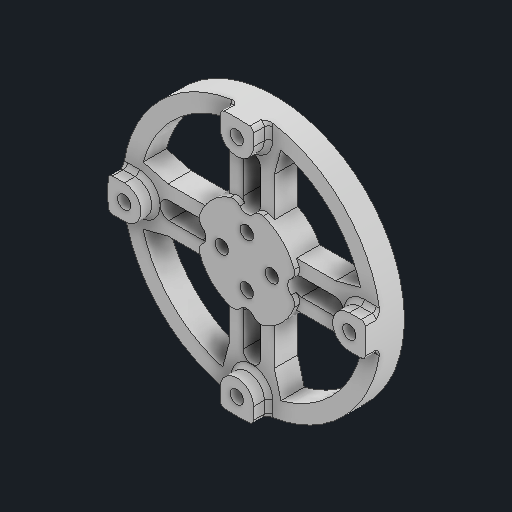
# Autodesk Inventor part: Rotator_B
Saved by Autodesk Inventor 2025.1 (Build 291241020, 241B)
## iProperties
Created: 2025-07-24
Part Number: Rotator_B
Material: 일반
Document SubType Name: Modeling
Designer: acalo
Density: 1 g/cm^3
Appearance: 기본값
Author: acalo
Autodesk Inventor part; units mm, degrees
ref_plane "YZ Plane" through (0, 0, 0) normal (1, 0, 0) x (0, 1, 0)
ref_plane "XZ Plane" through (0, 0, 0) normal (0, 1, 0) x (-1, 0, 0)
ref_plane "XY Plane" through (0, 0, 0) normal (0, 0, 1) x (1, 0, 0)
sketch "스케치1" plane through (0, 0, 0) normal (0, 0, 1) x (1, 0, 0)
  circle A0 centre (27, 0) radius 1.65
  circle A1 centre (0, 0) radius 31
  line L0 (5.4, 20.1531) -> (6.9881, 26.08)
  line L1 (20.1531, 5.4) -> (26.08, 6.9881)
  arc A2 (26.08, 6.9881) -> (6.9881, 26.08) centre (0, 0) ccw
  circle A3 centre (-4.8, 0) radius 1.65
  circle A4 centre (4.8, 0) radius 1.65
  line L2 (-5.4, 20.1531) -> (-6.9881, 26.08)
  line L3 (-20.1531, 5.4) -> (-26.08, 6.9881)
  arc A5 (-6.9881, 26.08) -> (-26.08, 6.9881) centre (0, 0) ccw
  line L4 (5.4, -20.1531) -> (6.9881, -26.08)
  line L5 (20.1531, -5.4) -> (26.08, -6.9881)
  arc A6 (6.9881, -26.08) -> (26.08, -6.9881) centre (0, 0) ccw
  line L6 (-20.1531, -5.4) -> (-26.08, -6.9881)
  arc A7 (-26.08, -6.9881) -> (-6.9881, -26.08) centre (0, 0) ccw
  line L7 (-5.4, -20.1531) -> (-6.9881, -26.08)
  line L8 (20.1531, -5.4) -> (8.4167, -5.4)
  line L9 (5.4, -8.4167) -> (5.4, -20.1531)
  line L10 (-5.4, -8.4167) -> (-5.4, -20.1531)
  line L11 (-8.4167, -5.4) -> (-20.1531, -5.4)
  line L12 (-5.4, 20.1531) -> (-5.4, 8.4167)
  line L13 (-8.4167, 5.4) -> (-20.1531, 5.4)
  line L14 (20.1531, 5.4) -> (8.4167, 5.4)
  line L15 (5.4, 20.1531) -> (5.4, 8.4167)
  arc A8 (-5.4, 8.4167) -> (-8.4167, 5.4) centre (0, 0) ccw
  arc A9 (8.4167, 5.4) -> (5.4, 8.4167) centre (0, 0) ccw
  arc A10 (-8.4167, -5.4) -> (-5.4, -8.4167) centre (0, 0) ccw
  arc A11 (5.4, -8.4167) -> (8.4167, -5.4) centre (0, 0) ccw
  circle A12 centre (0, 27) radius 1.65
  circle A13 centre (-27, 0) radius 1.65
  circle A14 centre (0, -27) radius 1.65
  line L16 (-27, 0) -> (-4.8, 0)
  line L17 (-19.9, 0) -> (-11.9, 0) construction
  line L18 (-19.9, -2.1) -> (-11.9, -2.1)
  line L19 (-11.9, 2.1) -> (-19.9, 2.1)
  arc A15 (-19.9, 2.1) -> (-19.9, -2.1) centre (-19.9, 0) ccw
  arc A16 (-11.9, -2.1) -> (-11.9, 2.1) centre (-11.9, 0) ccw
  arc A17 (2.1, -11.9) -> (-2.1, -11.9) centre (0, -11.9) ccw
  line L20 (2.1, -19.9) -> (2.1, -11.9)
  line L21 (0, -19.9) -> (0, -11.9) construction
  line L22 (-2.1, -11.9) -> (-2.1, -19.9)
  line L23 (0, -27) -> (0, -4.8)
  arc A18 (-2.1, -19.9) -> (2.1, -19.9) centre (0, -19.9) ccw
  arc A19 (11.9, 2.1) -> (11.9, -2.1) centre (11.9, 0) ccw
  line L24 (19.9, 2.1) -> (11.9, 2.1)
  line L25 (19.9, 0) -> (11.9, 0) construction
  line L26 (11.9, -2.1) -> (19.9, -2.1)
  line L27 (27, 0) -> (4.8, 0)
  arc A20 (19.9, -2.1) -> (19.9, 2.1) centre (19.9, 0) ccw
  arc A21 (-2.1, 11.9) -> (2.1, 11.9) centre (0, 11.9) ccw
  line L28 (-2.1, 19.9) -> (-2.1, 11.9)
  line L29 (0, 19.9) -> (0, 11.9) construction
  line L30 (2.1, 11.9) -> (2.1, 19.9)
  line L31 (0, 27) -> (0, 4.8)
  arc A22 (2.1, 19.9) -> (-2.1, 19.9) centre (0, 19.9) ccw
  circle A23 centre (0, 0) radius 12
  point P0 (5.9528, 22.2163)
  point P1 (22.2163, 5.9528)
  point P2 (-5.9528, 22.2163)
  point P3 (-22.2163, 5.9528)
  point P4 (5.9528, -22.2163)
  point P5 (22.2163, -5.9528)
  point P6 (-22.2163, -5.9528)
  point P7 (-5.9528, -22.2163)
  point P8 (-15.9, 0)
  point P9 (0, -15.9)
  point P10 (15.9, 0)
  point P11 (0, 15.9)
  point P12 (11.8151, 2.0983)
  point P13 (2.0983, 11.8151)
  point P14 (-2.0983, 11.8151)
  point P15 (-11.8151, 2.0983)
  point P16 (-11.8151, -2.0983)
  point P17 (-2.0983, -11.8151)
  point P18 (2.0983, -11.8151)
  point P19 (11.8151, -2.0983)
  point P20 (5.4, 10.7163)
  point P21 (10.7163, 5.4)
  point P22 (10.7163, -5.4)
  point P23 (5.4, -10.7163)
  point P24 (-5.4, -10.7163)
  point P25 (-10.7163, -5.4)
  point P26 (-10.7163, 5.4)
  point P27 (-5.4, 10.7163)
  dimension "d19" = 3.3
  dimension "d24" = 360
  dimension "d26" = 4
  dimension "d27" = 4.2
  dimension "d30" = 360
  dimension "d32" = 24
  constraints: 72 end point, 32 point on circle, 24 centre point, 12 point on line, 4 tangent, 3 horizontal, 2 coincident, 2 midpoint, 1 parallel, 70 other
  measures "d19" diameter of A4
  measures "d26" distance of point (-15.9, 0) L17.end
  measures "d27" diameter of A16
  measures "d32" diameter of A23
extrude "돌출1" add sketch "스케치1" along normal blind 4.8 contours A23 L14 A9 L15 | L15 A9 L14 A23 A19 L8 A11 L9 A17 L10 A10 L11 A16 L13 A8 L12 A21 | L12 A8 L13 A23 | A23 L9 A11 L8 | L11 A10 L10 A23
extrude "돌출2" add sketch "스케치1" along normal blind 3.6 contours A1
fillet "모깎기1" radius 2 8 edges at (2.0983, 11.8151, 4.2) (-2.0983, 11.8151, 4.2) (-11.8151, 2.0983, 4.2) (-11.8151, -2.0983, 4.2) (-2.0983, -11.8151, 4.2) (2.0983, -11.8151, 4.2) (11.8151, -2.0983, 4.2) (11.8151, 2.0983, 4.2)
sketch "스케치2" plane through (0, 0, 0) normal (0, 0, -1) x (-1, 0, 0)
  arc A0 (-2.1, 11.9) -> (2.1, 11.9) centre (0, 11.9) ccw projected
  line L0 (-2.1, 19.9) -> (-2.1, 11.9) projected
  arc A1 (2.1, 19.9) -> (-2.1, 19.9) centre (0, 19.9) ccw projected
  line L1 (2.1, 11.9) -> (2.1, 19.9) projected
  line L2 (5.4, 20.1531) -> (5.4, 10.7163) projected
  line L3 (6.9881, 26.08) -> (5.4, 20.1531) projected
  arc A2 (26.08, 6.9881) -> (6.9881, 26.08) centre (0, 0) ccw projected
  line L4 (20.1531, 5.4) -> (26.08, 6.9881) projected
  line L5 (10.7163, 5.4) -> (20.1531, 5.4) projected
  arc A3 (10.7163, 5.4) -> (5.4, 10.7163) centre (0, 0) ccw projected
  arc A4 (11.9, 2.1) -> (11.9, -2.1) centre (11.9, 0) ccw projected
  line L6 (19.9, 2.1) -> (11.9, 2.1) projected
  arc A5 (19.9, -2.1) -> (19.9, 2.1) centre (19.9, 0) ccw projected
  line L7 (11.9, -2.1) -> (19.9, -2.1) projected
  line L8 (20.1531, -5.4) -> (10.7163, -5.4) projected
  line L9 (26.08, -6.9881) -> (20.1531, -5.4) projected
  arc A6 (6.9881, -26.08) -> (26.08, -6.9881) centre (0, 0) ccw projected
  line L10 (5.4, -20.1531) -> (6.9881, -26.08) projected
  line L11 (5.4, -10.7163) -> (5.4, -20.1531) projected
  arc A7 (5.4, -10.7163) -> (10.7163, -5.4) centre (0, 0) ccw projected
  arc A8 (2.1, -11.9) -> (-2.1, -11.9) centre (0, -11.9) ccw projected
  line L12 (2.1, -19.9) -> (2.1, -11.9) projected
  arc A9 (-2.1, -19.9) -> (2.1, -19.9) centre (0, -19.9) ccw projected
  line L13 (-2.1, -11.9) -> (-2.1, -19.9) projected
  line L14 (-5.4, -20.1531) -> (-5.4, -10.7163) projected
  line L15 (-6.9881, -26.08) -> (-5.4, -20.1531) projected
  arc A10 (-26.08, -6.9881) -> (-6.9881, -26.08) centre (0, 0) ccw projected
  line L16 (-20.1531, -5.4) -> (-26.08, -6.9881) projected
  line L17 (-10.7163, -5.4) -> (-20.1531, -5.4) projected
  arc A11 (-10.7163, -5.4) -> (-5.4, -10.7163) centre (0, 0) ccw projected
  arc A12 (-11.9, -2.1) -> (-11.9, 2.1) centre (-11.9, 0) ccw projected
  line L18 (-19.9, -2.1) -> (-11.9, -2.1) projected
  arc A13 (-19.9, 2.1) -> (-19.9, -2.1) centre (-19.9, 0) ccw projected
  line L19 (-11.9, 2.1) -> (-19.9, 2.1) projected
  circle A14 centre (-27, 0) radius 1.65 projected
  circle A15 centre (0, -27) radius 1.65 projected
  circle A16 centre (27, 0) radius 1.65 projected
  circle A17 centre (0, 27) radius 1.65 projected
  circle A18 centre (0, 0) radius 31 projected
  line L20 (-20.1531, 5.4) -> (-10.7163, 5.4) projected
  line L21 (-26.08, 6.9881) -> (-20.1531, 5.4) projected
  arc A19 (-6.9881, 26.08) -> (-26.08, 6.9881) centre (0, 0) ccw projected
  line L22 (-5.4, 20.1531) -> (-6.9881, 26.08) projected
  line L23 (-5.4, 10.7163) -> (-5.4, 20.1531) projected
  arc A20 (-5.4, 10.7163) -> (-10.7163, 5.4) centre (0, 0) ccw projected
  circle A21 centre (-4.8, 0) radius 1.65 projected
  circle A22 centre (4.8, 0) radius 1.65 projected
  circle A23 centre (0, -27) radius 2.8
  circle A24 centre (-27, 0) radius 2.8
  circle A25 centre (0, 27) radius 2.8
  circle A26 centre (27, 0) radius 2.8
  dimension "d38" = 5.6
  dimension "d39" = 5.6
  dimension "d40" = 5.6
  dimension "d41" = 5.6
  constraints: 4 centre point, 1 coincident
  measures "d38" diameter of A23
  measures "d39" diameter of A24
  measures "d40" diameter of A25
  measures "d41" diameter of A26
sketch "스케치3" plane through (0, 0, 3.6) normal (0, 0, 1) x (1, 0, 0)
  circle A0 centre (0, -27) radius 1.65 projected
  circle A1 centre (0, 0) radius 31 projected
  arc A2 (4, -27) -> (-4, -27) centre (0, -27) ccw
  line L0 (-4, -27) -> (-4, -30.7409)
  line L1 (0, -27) -> (0, -16.0114)
  line L2 (4, -27) -> (4, -30.7409)
  constraints: 6 end point, 4 point on circle, 3 vertical, 1 centre point, 1 coincident, 1 tangent
extrude "돌출4" add sketch "스케치3" along normal blind 3.6 contours L0 A2 L2 A1 picked at (3.1504, -28.5087)
pattern_circular "원형 패턴1" count 4 over 360 about axis through (0, 0, 0) along (0, 0, 1) of "돌출4"
fillet "모깎기2" radius 1 8 edges at (-4, -30.7409, 5.4) (4, -30.7409, 5.4) (30.7409, -4, 5.4) (30.7409, 4, 5.4) (4, 30.7409, 5.4) (-4, 30.7409, 5.4) (-30.7409, 4, 5.4) (-30.7409, -4, 5.4)
fillet "모깎기3" radius 1 20 edges at (23, 0, 3.6) (28.4248, 4, 3.6) (30.5204, 3.7416, 3.6) (30.5204, -3.7416, 3.6) (28.4248, -4, 3.6) (3.7416, -30.5204, 3.6) (0, -23, 3.6) (-4, -28.4248, 3.6) (-3.7416, -30.5204, 3.6) (4, -28.4248, 3.6) (-4, 28.4248, 3.6) (-3.7416, 30.5204, 3.6) (4, 28.4248, 3.6) (3.7416, 30.5204, 3.6) (0, 23, 3.6) (-28.4248, -4, 3.6) (-30.5204, -3.7416, 3.6) (-28.4248, 4, 3.6) (-30.5204, 3.7416, 3.6) (-23, 0, 3.6)
thicken "두껍게 하기1" operation add thickness 2 both sides no extend neighbours no toward (0, 0, -1) faces at (0.0844, 4.0012, 0)
sketch "스케치4" plane through (0, 0, 4.8) normal (0, 0, 1) x (1, 0, 0)
  circle A0 centre (0, 0) radius 10
  circle A1 centre (4.8, 0) radius 1.65 projected
  circle A2 centre (-4.8, 0) radius 1.65 projected
  line L0 (0, 0) -> (0, 6)
  circle A3 centre (0, 6) radius 1.65
  line L1 (0, 6) -> (0, 8.7)
  line L2 (1.5588, 8.7) -> (3.1177, 6)
  line L3 (3.1177, 6) -> (1.5588, 3.3)
  line L4 (1.5588, 3.3) -> (-1.5588, 3.3)
  line L5 (-1.5588, 3.3) -> (-3.1177, 6)
  line L6 (-3.1177, 6) -> (-1.5588, 8.7)
  line L7 (-1.5588, 8.7) -> (1.5588, 8.7)
  circle A4 centre (-6, 0) radius 1.65
  line L8 (-6, 3.1177) -> (-3.3, 1.5588)
  line L9 (-3.3, 1.5588) -> (-3.3, -1.5588)
  line L10 (-3.3, -1.5588) -> (-6, -3.1177)
  line L11 (-6, -3.1177) -> (-8.7, -1.5588)
  line L12 (-8.7, -1.5588) -> (-8.7, 1.5588)
  line L13 (-8.7, 1.5588) -> (-6, 3.1177)
  circle A5 centre (0, -6) radius 1.65
  line L14 (-3.1177, -6) -> (-1.5588, -3.3)
  line L15 (-1.5588, -3.3) -> (1.5588, -3.3)
  line L16 (1.5588, -3.3) -> (3.1177, -6)
  line L17 (3.1177, -6) -> (1.5588, -8.7)
  line L18 (1.5588, -8.7) -> (-1.5588, -8.7)
  line L19 (-1.5588, -8.7) -> (-3.1177, -6)
  circle A6 centre (6, 0) radius 1.65
  line L20 (6, -3.1177) -> (3.3, -1.5588)
  line L21 (3.3, -1.5588) -> (3.3, 1.5588)
  line L22 (3.3, 1.5588) -> (6, 3.1177)
  line L23 (6, 3.1177) -> (8.7, 1.5588)
  line L24 (8.7, 1.5588) -> (8.7, -1.5588)
  line L25 (8.7, -1.5588) -> (6, -3.1177)
  point P0 (-8.7, 0)
  point P1 (0, -8.7)
  point P2 (8.7, 0)
  point P3 (-3.3, -0.6874)
  point P4 (-3.3, 0.6874)
  dimension "d53" = 20
  dimension "d54" = 6
  dimension "d55" = 3.3
  dimension "d56" = 2.7
  dimension "d59" = 360
  constraints: 52 end point, 5 centre point, 3 coincident, 2 vertical, 1 midpoint, 74 other
  measures "d53" diameter of A0
  measures "d54" distance of L0.start L0.end
  measures "d55" diameter of A3
  measures "d56" distance of L1.start L1.end
extrude "돌출5" add sketch "스케치4" against normal up to surface (6.8 mm away) contours A1 A6 | A6 A1 L21 | L21 A1 | A2 L9 | L9 A2 A4 | A4 A2 picked at (5.0657, -0.1306) picked at (-5.0657, 0.1306)
extrude "돌출6" cut sketch "스케치4" against normal through all contours A1 A6 | A1 A6 | A4 A2 | A2 A4 | A3 L1 L0 | L0 L1 A3 | A5
sketch "스케치5" plane through (0, 0, 4.8) normal (0, 0, 1) x (1, 0, 0)
  circle A0 centre (0, -6) radius 1.65 projected
  circle A1 centre (0, -6) radius 1.6
  point P0 (0, 0)
  dimension "d65" = 3.2
  constraints: 1 centre point, 1 coincident
  measures "d65" diameter of A1
extrude "돌출7" add sketch "스케치5" against normal up to surface (6.8 mm away)
sketch "스케치6" plane through (0, 0, 7.2) normal (0, 0, 1) x (1, 0, 0)
  circle A0 centre (0, -27) radius 1.65 projected
  circle A1 centre (0, -27) radius 1.6
  point P0 (0, 0)
  dimension "d68" = 0.05
  constraints: 1 centre point
  measures "d68" radial gap between concentric circles of A0 A1
extrude "돌출8" add sketch "스케치6" against normal up to surface (9.2 mm away)
pattern_circular "원형 패턴2" count 4 over 360 about axis through (0, 0, 0) along (0, 0, 1) of "돌출7", "돌출8"
sketch "스케치7" plane through (0, 0, -2) normal (0, 0, -1) x (-1, 0, 0)
  circle A0 centre (0, 27) radius 1.6 projected
  circle A1 centre (6, 0) radius 1.6 projected
  circle A2 centre (27, 0) radius 1.6 projected
  circle A3 centre (0, 6) radius 1.6 projected
  circle A4 centre (0, 27) radius 1.6 projected
  circle A5 centre (-6, 0) radius 1.6 projected
  circle A6 centre (-27, 0) radius 1.6 projected
  circle A7 centre (0, -27) radius 1.6 projected
  circle A8 centre (0, -6) radius 1.6 projected
  line L0 (-20.1531, 5.4) -> (-10.7163, 5.4) projected
  line L1 (-26.08, 6.9881) -> (-20.1531, 5.4) projected
  arc A9 (-6.9881, 26.08) -> (-26.08, 6.9881) centre (0, 0) ccw projected
  line L2 (-5.4, 20.1531) -> (-6.9881, 26.08) projected
  line L3 (-5.4, 10.7163) -> (-5.4, 20.1531) projected
  arc A10 (-5.4, 10.7163) -> (-10.7163, 5.4) centre (0, 0) ccw projected
  circle A11 centre (0, 0) radius 31 projected
  arc A12 (-11.9, -2.1) -> (-11.9, 2.1) centre (-11.9, 0) ccw projected
  line L4 (-19.9, -2.1) -> (-11.9, -2.1) projected
  arc A13 (-19.9, 2.1) -> (-19.9, -2.1) centre (-19.9, 0) ccw projected
  line L5 (-11.9, 2.1) -> (-19.9, 2.1) projected
  line L6 (-5.4, -20.1531) -> (-5.4, -10.7163) projected
  line L7 (-6.9881, -26.08) -> (-5.4, -20.1531) projected
  arc A14 (-26.08, -6.9881) -> (-6.9881, -26.08) centre (0, 0) ccw projected
  line L8 (-20.1531, -5.4) -> (-26.08, -6.9881) projected
  line L9 (-10.7163, -5.4) -> (-20.1531, -5.4) projected
  arc A15 (-10.7163, -5.4) -> (-5.4, -10.7163) centre (0, 0) ccw projected
  arc A16 (2.1, -11.9) -> (-2.1, -11.9) centre (0, -11.9) ccw projected
  line L10 (2.1, -19.9) -> (2.1, -11.9) projected
  arc A17 (-2.1, -19.9) -> (2.1, -19.9) centre (0, -19.9) ccw projected
  line L11 (-2.1, -11.9) -> (-2.1, -19.9) projected
  line L12 (20.1531, -5.4) -> (10.7163, -5.4) projected
  line L13 (26.08, -6.9881) -> (20.1531, -5.4) projected
  arc A18 (6.9881, -26.08) -> (26.08, -6.9881) centre (0, 0) ccw projected
  line L14 (5.4, -20.1531) -> (6.9881, -26.08) projected
  line L15 (5.4, -10.7163) -> (5.4, -20.1531) projected
  arc A19 (5.4, -10.7163) -> (10.7163, -5.4) centre (0, 0) ccw projected
  arc A20 (11.9, 2.1) -> (11.9, -2.1) centre (11.9, 0) ccw projected
  line L16 (19.9, 2.1) -> (11.9, 2.1) projected
  arc A21 (19.9, -2.1) -> (19.9, 2.1) centre (19.9, 0) ccw projected
  line L17 (11.9, -2.1) -> (19.9, -2.1) projected
  line L18 (5.4, 20.1531) -> (5.4, 10.7163) projected
  line L19 (6.9881, 26.08) -> (5.4, 20.1531) projected
  arc A22 (26.08, 6.9881) -> (6.9881, 26.08) centre (0, 0) ccw projected
  line L20 (20.1531, 5.4) -> (26.08, 6.9881) projected
  line L21 (10.7163, 5.4) -> (20.1531, 5.4) projected
  arc A23 (10.7163, 5.4) -> (5.4, 10.7163) centre (0, 0) ccw projected
  arc A24 (-2.1, 11.9) -> (2.1, 11.9) centre (0, 11.9) ccw projected
  line L22 (-2.1, 19.9) -> (-2.1, 11.9) projected
  arc A25 (2.1, 19.9) -> (-2.1, 19.9) centre (0, 19.9) ccw projected
  line L23 (2.1, 11.9) -> (2.1, 19.9) projected
  circle A26 centre (0, 27) radius 2.8
  circle A27 centre (27, 0) radius 2.8
  circle A28 centre (0, -27) radius 2.8
  circle A29 centre (-27, 0) radius 2.8
  dimension "d74" = 5.6
  dimension "d75" = 5.6
  dimension "d76" = 5.6
  dimension "d77" = 5.6
  constraints: 4 centre point, 1 coincident
  measures "d74" diameter of A26
  measures "d75" diameter of A27
  measures "d76" diameter of A28
  measures "d77" diameter of A29
extrude "돌출9" cut sketch "스케치7" against normal blind 2 contours A0 | A2 | A6 | A7 | A26 | A27 | A28 | A29
